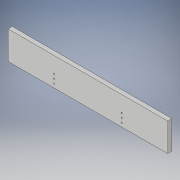
# Autodesk Inventor part: Long Plank
Saved by Autodesk Inventor 2018 (Build 220112000, 112)
## iProperties
Created: 2020-01-22
Part Number: Long Plank
Material: Generic
Document SubType Name: Modeling
Designer: s-2512711
Density: 1 g/cm^3
Appearance: Default
Author: s-2512711
Autodesk Inventor part; units mm, degrees
ref_plane "YZ Plane" through (0, 0, 0) normal (1, 0, 0) x (0, 1, 0)
ref_plane "XZ Plane" through (0, 0, 0) normal (0, 1, 0) x (-1, 0, 0)
ref_plane "XY Plane" through (0, 0, 0) normal (0, 0, 1) x (1, 0, 0)
sketch "Sketch1" plane through (0, 0, 0) normal (0, 0, 1) x (1, 0, 0)
  line L0 (0, 0) -> (719.074, 0)
  line L1 (719.074, 0) -> (719.074, 127)
  line L2 (719.074, 127) -> (0, 127)
  line L3 (0, 127) -> (0, 0)
  dimension "d0" = 719.074
  dimension "d1" = 127
  constraints: 8 end point, 2 parallel, 1 horizontal, 1 perpendicular
  measures "d0" distance of L2.end L1.end
  measures "d1" distance of L1.end L0.end
extrude "Extrusion1" add sketch "Sketch1" along normal blind 19.05
sketch "Sketch2" plane through (0, 0, 19.05) normal (0, 0, 1) x (1, 0, 0)
  line L0 (0, 0) -> (719.074, 0) construction
  line L1 (0, 0) -> (207.137, 0) construction
  line L2 (207.137, 0) -> (207.137, 17.018) construction
  line L3 (207.137, 17.018) -> (207.137, 36.068) construction
  line L4 (207.137, 36.068) -> (207.137, 55.118) construction
  line L5 (719.074, 127) -> (0, 127) construction
  line L6 (359.537, 127) -> (359.537, 0) construction
  circle A0 centre (207.137, 17.018) radius 2.667
  circle A1 centre (207.137, 36.068) radius 2.667
  circle A2 centre (207.137, 55.118) radius 2.667
  line L7 (511.937, 17.018) -> (511.937, 36.068) construction
  line L8 (511.937, 36.068) -> (511.937, 55.118) construction
  circle A3 centre (511.937, 17.018) radius 2.667
  circle A4 centre (511.937, 36.068) radius 2.667
  circle A5 centre (511.937, 55.118) radius 2.667
  dimension "d4" = 207.137
  dimension "d5" = 17.018
  dimension "d6" = 19.05
  dimension "d7" = 19.05
  dimension "d8" = 5.334
  constraints: 14 end point, 6 centre point, 6 coincident, 6 symmetric about line, 4 point on line, 2 midpoint, 1 perpendicular, 3 other
  measures "d4" distance of L0.start L1.end
  measures "d5" distance of L1.end L2.end
  measures "d6" distance of L2.end L3.end
  measures "d7" distance of L3.end L4.end
  measures "d8" diameter of A0
extrude "Extrusion2" cut sketch "Sketch2" against normal blind 19.05
body "Solid1"
